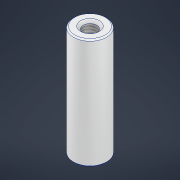
# Autodesk Inventor part: Spacer_M3D6L60
Saved by Autodesk Inventor 2022.4 (Build 264492010, 492A)
## iProperties
Created: 2022-02-26
Part Number: Spacer_M3D6L60
Material: アルミニウム 6061
Document SubType Name: Modeling
Designer: Yuta Fujiyama
Density: 2.7 g/cm^3
Appearance: アルミニウム - フラット
Author: Yuta Fujiyama
Autodesk Inventor part; units mm, degrees
ref_plane "YZ Plane" through (0, 0, 0) normal (1, 0, 0) x (0, 1, 0)
ref_plane "XZ Plane" through (0, 0, 0) normal (0, 1, 0) x (-1, 0, 0)
ref_plane "XY Plane" through (0, 0, 0) normal (0, 0, 1) x (1, 0, 0)
sketch "スケッチ1" plane through (0, 0, 0) normal (0, 1, 0) x (-1, 0, 0)
  circle A0 centre (0, 0) radius 3
  dimension "d0" = 6
  constraints: 1 centre point, 1 coincident
  measures "d0" diameter of A0
extrude "押し出し1" add sketch "スケッチ1" along normal mid plane 20
sketch "スケッチ2" plane through (0, 10, 0) normal (0, 1, 0) x (1, 0, 0)
  point P0 (0, 0)
  point P1 (0, 0)
  constraints: 1 coincident
hole "穴1" at (0, 10, 0) direction (0, -1, 0) diameter 2.459 depth 10 countersink diameter 3.4 countersink angle 90 thread size "M3x0.5" class "6H" standard "ISO Metric profile"
sketch "スケッチ3" plane through (0, -10, 0) normal (0, -1, 0) x (1, 0, 0)
  point P0 (0, 0)
  point P1 (0, 0)
  constraints: 1 coincident
hole "穴2" at (0, -10, 0) direction (0, 1, 0) diameter 2.459 depth 10 countersink diameter 3.4 countersink angle 90 thread size "M3x0.5" class "6H" standard "ISO Metric profile"
chamfer "面取り1" distance 0.25 angle 45 2 edges at (3, -10, 0) (3, 10, 0)
